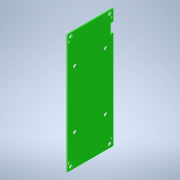
# Autodesk Inventor part: SolarPCB_RBF_EGSE
Saved by Autodesk Inventor 2022 (Build 260153000, 153)
## iProperties
Created: 2021-09-09
Part Number: SolarPCB_RBF_EGSE
Material: Acetal Resin, Black
Document SubType Name: Modeling
Designer: Bowen O'Steen
Density: 1.425 g/cm^3
Appearance: Dark Green
Author: Bowen O'Steen
Autodesk Inventor part; units mm, degrees
ref_plane "YZ Plane" through (0, 0, 0) normal (1, 0, 0) x (0, 1, 0)
ref_plane "XZ Plane" through (0, 0, 0) normal (0, 1, 0) x (-1, 0, 0)
ref_plane "XY Plane" through (0, 0, 0) normal (0, 0, 1) x (1, 0, 0)
sketch "Sketch1" plane through (0, 0, 0) normal (1, 0, 0) x (0, 1, 0)
  line L0 (50, 41.5) -> (-50, 41.5)
  line L1 (-50, 41.5) -> (-50, -41.5)
  line L2 (-50, -41.5) -> (50, -41.5)
  line L3 (50, -41.5) -> (50, 41.5)
  point P0 (0, 0)
  point P1 (50, 0)
  point P2 (0, -41.5)
  dimension "d0" = 100
  dimension "d1" = 83
  constraints: 8 end point, 2 midpoint, 2 parallel, 1 horizontal, 1 horizontal alignment, 1 perpendicular, 1 vertical alignment
  measures "d0" distance of L1.end L2.end
  measures "d1" distance of L2.end L0.start
extrude "Extrusion1" add sketch "Sketch1" along normal blind 1.6
sketch "Sketch12" plane through (0, 50, 41.5) normal (0, 1, 0) x (1, 0, 0)
  line L0 (0, 83) -> (0, 0) projected
  line L1 (0, 0) -> (1.6, 0) projected
  line L2 (1.6, 83) -> (1.6, 0) projected
  line L3 (0, 83) -> (1.6, 83) projected
  point P0 (0, 41.5)
extrude "Extrusion3" add sketch "Sketch12" along normal blind 56.75
sketch "Sketch13" plane through (0, -50, -41.5) normal (0, -1, 0) x (1, 0, 0)
  line L0 (0, 83) -> (0, 0) projected
  line L1 (0, 0) -> (1.6, 0) projected
  line L2 (1.6, 83) -> (1.6, 0) projected
  line L3 (0, 83) -> (1.6, 83) projected
  point P0 (0, 41.5)
extrude "Extrusion4" add sketch "Sketch13" along normal blind 56.75
sketch "Sketch14" plane through (0, 0, 0) normal (-1, 0, 0) x (0, 0, 1)
  point P0 (0, 0)
  point P1 (27.5, -51.25)
  point P2 (27.5, 51.25)
  point P3 (-27.5, -51.25)
  point P4 (-27.5, 51.25)
  dimension "d156" = 102.5
  dimension "d157" = 102.5
  dimension "d158" = 55
  dimension "d159" = 27.5
  dimension "d160" = 51.25
  constraints: 2 vertical alignment, 1 horizontal alignment
  measures "d156" distance of point (27.5, 51.25) point (27.5, -51.25)
  measures "d157" distance of point (-27.5, 51.25) point (-27.5, -51.25)
  measures "d158" distance of point (27.5, -51.25) point (-27.5, -51.25)
  measures "d159" horizontal distance of point (-27.5, -51.25) point (0, 0)
  measures "d160" vertical distance of point (0, 0) point (-27.5, -51.25)
hole "Hole7" at (0, -51.25, 27.5) at (0, 51.25, 27.5) at (0, -51.25, -27.5) at (0, 51.25, -27.5) direction (1, 0, 0) diameter 6 end through all
sketch "Sketch16" plane through (0, 0, 0) normal (-1, 0, 0) x (0, 0, 1)
  circle A0 centre (-27.5, -51.25) radius 3 projected
  circle A1 centre (27.5, -51.25) radius 3 projected
  circle A2 centre (27.5, 51.25) radius 3 projected
  circle A3 centre (-27.5, 51.25) radius 3 projected
  line L0 (41.5, -106.75) -> (41.5, 106.75) projected
  line L1 (-41.5, 106.75) -> (41.5, 106.75) projected
  line L2 (-41.5, 106.75) -> (-41.5, -106.75) projected
  line L3 (41.5, -106.75) -> (-41.5, -106.75) projected
  line L4 (0, 0) -> (-25, 0) construction
  point P0 (35, -100.75)
  point P1 (-35, -100.75)
  point P2 (35, 100.75)
  point P3 (-35, 100.75)
  dimension "d168" = 70
  dimension "d169" = 6
  dimension "d170" = 35
  constraints: 2 end point, 2 symmetric about line, 1 horizontal, 1 horizontal alignment
  measures "d168" distance of point (-35, -100.75) point (35, -100.75)
  measures "d169" distance from line of L3 point (35, -100.75)
  measures "d170" horizontal distance of L4.start point (-35, -100.75)
hole "Hole8" at (0, -100.75, 35) at (0, -100.75, -35) at (0, 100.75, 35) at (0, 100.75, -35) direction (1, 0, 0) diameter 6 end through all
sketch "Sketch19" plane through (0, 0, 0) normal (-1, 0, 0) x (0, 0, 1)
  circle A0 centre (-27.5, 51.25) radius 3 construction
  line L0 (-39, 76.75) -> (-39, 72) construction
  line L1 (-39, 76.75) -> (-39, 81.5) construction
  line L2 (-41.5, 106.75) -> (-41.5, -106.75) construction
  line L3 (-41.5, 106.75) -> (41.5, 106.75) projected
  point P0 (0, 0)
  dimension "d194" = 4.75
  dimension "d195" = 4.75
  dimension "d203" = 25.25
  dimension "d204" = 2.5
  constraints: 4 end point, 2 coincident, 1 parallel, 1 vertical alignment
  measures "d194" distance of L0.start L0.end
  measures "d195" distance of L0.start L1.end
  measures "d203" distance from line of L3 point (-39, 81.5)
  measures "d204" distance from line of L2 point (-39, 81.5)
hole "Hole9" at (0, 72, -39) at (0, 81.5, -39) direction (1, 0, 0) diameter 2.6 end through all clearance for "Flat Head Machine Screw" size "M2" standard "Ansi Metric M Profile"
sketch "Sketch21" plane through (0, 0, 0) normal (-1, 0, 0) x (0, 0, 1)
  line L0 (-41.5, 106.75) -> (-41.5, -106.75) projected
  line L1 (-41.5, 85.75) -> (-36.5, 85.75)
  line L2 (-36.5, 85.75) -> (-36.5, 67.75)
  line L3 (-36.5, 67.75) -> (-41.5, 67.75)
  line L4 (-41.5, 67.75) -> (-41.5, 85.75)
  line L5 (-41.5, 106.75) -> (41.5, 106.75) projected
  point P0 (0, 0)
  point P1 (-41.5, 67.75)
  dimension "d205" = 5
  dimension "d206" = 21
  dimension "d207" = 18
  constraints: 8 end point, 2 parallel, 1 horizontal, 1 perpendicular, 1 point on line
  measures "d205" distance of L2.end L3.end
  measures "d206" distance between parallel lines of L5 L1
  measures "d207" distance of L1.end L2.end
extrude "Extrusion5" cut sketch "Sketch21" against normal through all
sketch "Sketch23" plane through (0, 0, 0) normal (-1, 0, 0) x (0, 0, 1)
  circle A0 centre (-35, 100.75) radius 3 projected
  line L0 (0, 0) -> (-12.2775, 0) construction
  point P0 (38, 93.75)
  point P1 (-38, 93.75)
  point P2 (38, -93.75)
  point P3 (-38, -93.75)
  dimension "d220" = 76
  dimension "d221" = 38
  dimension "d229" = 7
  constraints: 2 end point, 2 symmetric about line, 1 horizontal, 1 horizontal alignment
  measures "d220" distance of point (-38, 93.75) point (38, 93.75)
  measures "d221" horizontal distance of L0.start point (-38, 93.75)
  measures "d229" vertical distance of point (-38, 93.75) A0.centre
hole "Hole11" at (0, 93.75, 38) at (0, 93.75, -38) at (0, -93.75, 38) at (0, -93.75, -38) direction (1, 0, 0) diameter 3.454 end through all clearance for "Flat Head Machine Screw (82)" size "#4" standard "Ansi Unified Screw Threads"
equation "\"d157\" = d156"
equation "\"d159\" = 0.5 * d158"
equation "\"d160\" = 0.5 * d157"
equation "\"d170\" = 0.5 * d168"
equation "\"d195\" = d194"
equation "\"d221\" = 0.5 * d220"
body "Solid1"
